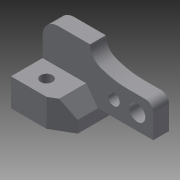
# Autodesk Inventor part: HW 8 Part 3
Saved by Autodesk Inventor 2015 SP1 (Build 190203100, 203)
## iProperties
Created: 2016-03-08
Part Number: HW 8 Part 3
Material: Generic
Document SubType Name: Modeling
Designer: Melissa
Density: 1 g/cm^3
Appearance: Default
Author: Melissa
Autodesk Inventor part; units mm, degrees
ref_plane "YZ Plane" through (0, 0, 0) normal (1, 0, 0) x (0, 1, 0)
ref_plane "XZ Plane" through (0, 0, 0) normal (0, 1, 0) x (-1, 0, 0)
ref_plane "XY Plane" through (0, 0, 0) normal (0, 0, 1) x (1, 0, 0)
sketch "Sketch1" plane through (0, 0, 0) normal (0, 0, 1) x (1, 0, 0)
  line L0 (0, 0) -> (0, 44.45)
  line L1 (0, 44.45) -> (69.85, 44.45)
  line L2 (69.85, 44.45) -> (88.9, 19.05)
  line L3 (88.9, 19.05) -> (88.9, 0)
  line L4 (88.9, 0) -> (0, 0)
  dimension "d0" = 44.45
  dimension "d1" = 69.85
  dimension "d2" = 88.9
  dimension "d3" = 19.05
  constraints: 10 end point, 2 perpendicular, 1 parallel, 1 vertical
  measures "d0" distance of L0.start L0.end
  measures "d1" distance of L0.end L1.end
  measures "d2" distance of L3.end L0.start
  measures "d3" distance of L2.end L3.end
extrude "Extrusion1" add sketch "Sketch1" against normal blind 76.2
sketch "Sketch2" plane through (0, 0, -76.2) normal (0, 0, -1) x (-1, 0, 0)
  line L0 (0, 0) -> (0, 19.05)
  line L1 (0, 0) -> (0, 44.45) projected
  line L2 (0, 19.05) -> (0, 76.2)
  line L3 (-25.4, 101.6) -> (-76.2, 101.6)
  line L4 (0, 19.05) -> (-177.8, 19.05)
  line L5 (-177.8, 19.05) -> (-177.8, 57.1575)
  arc A0 (-164.6625, 69.85) -> (-177.8, 57.1575) centre (-165.1, 57.1575) ccw
  arc A1 (0, 76.2) -> (-25.4, 101.6) centre (-25.4, 76.2) ccw
  line L6 (-164.6625, 69.85) -> (-136.9553, 69.85)
  arc A2 (-136.9553, 69.85) -> (-92.7612, 77.7875) centre (-136.9553, 196.85) ccw
  arc A3 (-92.7612, 77.7875) -> (-76.2, 101.6) centre (-101.6, 101.6) ccw
  point P0 (0, 101.6)
  dimension "d6" = 19.05
  dimension "d7" = 177.8
  dimension "d9" = 82.55
  dimension "d10" = 12.7
  dimension "d11" = 25.4
  dimension "d13" = 31.75
  dimension "d14" = 101.6
  dimension "d36" = 127
  dimension "d37" = 25.4
  constraints: 12 end point, 8 point on circle, 5 tangent, 4 centre point, 4 point on line, 2 horizontal, 2 perpendicular, 1 horizontal alignment
  measures "d6" distance of L0.start L0.end
  measures "d7" distance of L0.end L4.end
  measures "d9" distance of L0.end point (0, 101.6)
  measures "d10" radius of A0
  measures "d11" radius of A1
  measures "d13" vertical distance of L6.start L3.end
  measures "d14" horizontal distance of L4.end L3.end
  measures "d36" radius of A2
  measures "d37" radius of A3
extrude "Extrusion2" add sketch "Sketch2" against normal blind 25.4 separate body
sketch "Sketch3" plane through (0, 44.45, 0) normal (0, 1, 0) x (1, 0, 0)
  line L0 (0, 0) -> (57.15, 0)
  line L1 (0, 0) -> (69.85, 0) projected
  line L2 (57.15, 0) -> (106.8424, 28.6899)
  line L3 (106.8424, 28.6899) -> (106.8424, 0)
  line L4 (106.8424, 0) -> (57.15, 0)
  dimension "d18" = 57.15
  dimension "d19" = 30
  constraints: 8 end point, 2 perpendicular, 2 point on line
  measures "d18" distance of L0.start L0.end
  measures "d19" angle of L4 L2
extrude "Extrusion3" cut sketch "Sketch3" against normal through all bodies 1
sketch "Sketch4" plane through (0, 44.45, -76.2) normal (0, 1, 0) x (1, 0, 0)
  circle A0 centre (31.75, -50.8) radius 9.525
  line L0 (57.15, -76.2) -> (0, -76.2) projected
  line L1 (0, -76.2) -> (0, 0) projected
  dimension "d22" = 19.05
  dimension "d23" = 25.4
  dimension "d24" = 31.75
  constraints: 1 centre point
  measures "d22" diameter of A0
  measures "d23" distance from line of L0 A0.centre
  measures "d24" distance from line of L1 A0.centre
extrude "Extrusion4" cut sketch "Sketch4" against normal through all bodies 1
sketch "Sketch5" plane through (0, 0, -50.8) normal (0, 0, 1) x (1, 0, 0)
  circle A0 centre (152.4, 44.45) radius 12.7
  circle A1 centre (114.3, 44.45) radius 9.525
  line L0 (0, 19.05) -> (177.8, 19.05) projected
  line L1 (177.8, 19.05) -> (177.8, 57.1575) projected
  point P0 (0, 0)
  dimension "d27" = 25.4
  dimension "d28" = 19.05
  dimension "d29" = 25.4
  dimension "d30" = 38.1
  dimension "d32" = 25.4
  dimension "d33" = 0
  constraints: 2 centre point
  measures "d27" diameter of A0
  measures "d28" diameter of A1
  measures "d29" distance from line of L0 A1.centre
  measures "d30" distance of A0.centre A1.centre
  measures "d32" distance from line of L1 A0.centre
  measures "d33" vertical distance of A0.centre A1.centre
extrude "Extrusion5" cut sketch "Sketch5" against normal through all bodies 2
body "Solid1"
body "Solid2"
